# Autodesk Inventor part: C-channel 1
Saved by Autodesk Inventor 2014 (Build 180170000, 170)
## iProperties
Created: 2014-02-01
Part Number: C-channel 1
Material: Generic
Document SubType Name: Modeling
Designer: Alex
Density: 1 g/cm^3
Appearance: Default
Author: Alex
Autodesk Inventor part; units mm, degrees
ref_plane "YZ Plane" through (0, 0, 0) normal (1, 0, 0) x (0, 1, 0)
ref_plane "XZ Plane" through (0, 0, 0) normal (0, 1, 0) x (-1, 0, 0)
ref_plane "XY Plane" through (0, 0, 0) normal (0, 0, 1) x (1, 0, 0)
ref_plane "Work Plane1" through (0, 0, 0) normal (0, 0, 1) x (1, 0, 0)
sketch "Sketch1" plane through (0, 0, 0) normal (0, 0, 1) x (1, 0, 0)
  arc A0 (-113.2188, 0) -> (-109.7581, 3.4607) centre (-113.2188, 3.4607) ccw projected
  line L0 (-109.7581, 17.1767) -> (-109.7581, 3.4607) projected
  arc A1 (-109.7581, 17.1767) -> (-114.8063, 22.225) centre (-114.8063, 17.1767) ccw projected
  line L1 (-115.8223, 22.225) -> (-114.8063, 22.225) projected
  arc A2 (-115.8223, 22.225) -> (-119.2831, 18.7642) centre (-115.8223, 18.7642) ccw projected
  line L2 (-119.2831, 16.4211) -> (-119.2831, 18.7642) projected
  arc A3 (-119.2831, 16.4211) -> (-116.6161, 16.4211) centre (-117.9496, 16.4211) ccw projected
  line L3 (-116.6161, 18.7642) -> (-116.6161, 16.4211) projected
  arc A4 (-115.8223, 19.558) -> (-116.6161, 18.7642) centre (-115.8223, 18.7642) ccw projected
  line L4 (-114.8063, 19.558) -> (-115.8223, 19.558) projected
  arc A5 (-112.4251, 17.1767) -> (-114.8063, 19.558) centre (-114.8063, 17.1767) ccw projected
  line L5 (-112.4251, 3.4607) -> (-112.4251, 17.1767) projected
  arc A6 (-113.2188, 2.667) -> (-112.4251, 3.4607) centre (-113.2188, 3.4607) ccw projected
  line L6 (-147.5723, 2.667) -> (-113.2188, 2.667) projected
  arc A7 (-148.3661, 3.4607) -> (-147.5723, 2.667) centre (-147.5723, 3.4607) ccw projected
  line L7 (-148.3661, 17.1767) -> (-148.3661, 3.4607) projected
  arc A8 (-145.9848, 19.558) -> (-148.3661, 17.1767) centre (-145.9848, 17.1767) ccw projected
  line L8 (-144.9688, 19.558) -> (-145.9848, 19.558) projected
  arc A9 (-144.1751, 18.7642) -> (-144.9688, 19.558) centre (-144.9688, 18.7642) ccw projected
  line L9 (-144.1751, 16.4211) -> (-144.1751, 18.7642) projected
  arc A10 (-144.1751, 16.4211) -> (-141.5081, 16.4211) centre (-142.8416, 16.4211) ccw projected
  line L10 (-141.5081, 18.7642) -> (-141.5081, 16.4211) projected
  arc A11 (-141.5081, 18.7642) -> (-144.9688, 22.225) centre (-144.9688, 18.7642) ccw projected
  line L11 (-145.9848, 22.225) -> (-144.9688, 22.225) projected
  arc A12 (-145.9848, 22.225) -> (-151.0331, 17.1767) centre (-145.9848, 17.1767) ccw projected
  line L12 (-151.0331, 3.4607) -> (-151.0331, 17.1767) projected
  arc A13 (-151.0331, 3.4607) -> (-147.5723, 0) centre (-147.5723, 3.4607) ccw projected
  line L13 (-113.2188, 0) -> (-147.5723, 0) projected
  point P0 (0, 0)
extrude "Extrusion1" add sketch "Sketch1" along normal blind 796.925
body "Solid1"
